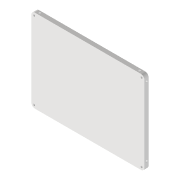
# Autodesk Inventor part: Omniscope_USBC_Illuminationunit
Saved by Autodesk Inventor 2022 (Build 260153000, 153)
## iProperties
Created: 2023-05-17
Part Number: Omniscope_USBC_Illuminationunit
Material: Generisch
Document SubType Name: Modeling
Designer: diederichbenedict
Density: 1 g/cm^3
Appearance: Vorgabe
Author: diederichbenedict
Autodesk Inventor part; units mm, degrees
ref_plane "YZ Plane" through (0, 0, 0) normal (1, 0, 0) x (0, 1, 0)
ref_plane "XZ Plane" through (0, 0, 0) normal (0, 1, 0) x (-1, 0, 0)
ref_plane "XY Plane" through (0, 0, 0) normal (0, 0, 1) x (1, 0, 0)
sketch "Skizze1" plane through (0, 0, 0) normal (0, 0, 1) x (1, 0, 0)
  line L0 (63.945, 39.8) -> (63.945, -39.8) construction
  arc A0 (63.945, 39.8) -> (60.945, 42.8) centre (60.945, 39.8) ccw construction
  line L1 (-60.945, 42.8) -> (60.945, 42.8) construction
  arc A1 (-60.945, 42.8) -> (-63.945, 39.8) centre (-60.945, 39.8) ccw construction
  line L2 (-63.945, -39.8) -> (-63.945, 39.8) construction
  arc A2 (-63.945, -39.8) -> (-60.945, -42.8) centre (-60.945, -39.8) ccw construction
  line L3 (60.945, -42.8) -> (-60.945, -42.8) construction
  arc A3 (60.945, -42.8) -> (63.945, -39.8) centre (60.945, -39.8) ccw construction
  line L4 (-63.625, -39.48) -> (-63.625, 39.48) construction
  arc A4 (-60.625, 42.48) -> (-63.625, 39.48) centre (-60.625, 39.48) ccw construction
  line L5 (-60.625, 42.48) -> (60.625, 42.48) construction
  arc A5 (63.625, 39.48) -> (60.625, 42.48) centre (60.625, 39.48) ccw construction
  line L6 (63.625, 39.48) -> (63.625, -39.48) construction
  arc A6 (60.625, -42.48) -> (63.625, -39.48) centre (60.625, -39.48) ccw construction
  line L7 (60.625, -42.48) -> (-60.625, -42.48) construction
  arc A7 (-63.625, -39.48) -> (-60.625, -42.48) centre (-60.625, -39.48) ccw construction
  line L8 (-62.625, 39.48) -> (-62.625, -39.48) construction
  arc A8 (-62.625, -39.48) -> (-60.625, -41.48) centre (-60.625, -39.48) ccw construction
  line L9 (-60.625, -41.48) -> (60.625, -41.48) construction
  arc A9 (60.625, -41.48) -> (62.625, -39.48) centre (60.625, -39.48) ccw construction
  line L10 (62.625, -39.48) -> (62.625, 39.48) construction
  arc A10 (62.625, 39.48) -> (60.625, 41.48) centre (60.625, 39.48) ccw construction
  line L11 (60.625, 41.48) -> (-60.625, 41.48) construction
  arc A11 (-60.625, 41.48) -> (-62.625, 39.48) centre (-60.625, 39.48) ccw construction
  line L12 (75.9176, 38) -> (78.9176, 41) construction
  line L13 (75.9176, 38) -> (66.9176, 38) construction
  line L14 (63.9176, 35) -> (66.9176, 38) construction
  line L15 (63.9176, 35) -> (63.9176, -34.9) construction
  line L16 (66.9176, -37.9) -> (63.9176, -34.9) construction
  line L17 (66.9176, -37.9) -> (75.9176, -37.9) construction
  line L18 (78.9176, -40.9) -> (75.9176, -37.9) construction
  line L19 (78.9176, -40.9) -> (78.9176, -45.7356) construction
  arc A12 (74.9176, -49.7356) -> (78.9176, -45.7356) centre (74.9176, -45.7356) ccw construction
  line L20 (74.9176, -49.7356) -> (-61.9244, -49.7356) construction
  arc A13 (-65.9244, -45.7356) -> (-61.9244, -49.7356) centre (-61.9244, -45.7356) ccw projected
  line L21 (-65.9244, -45.7356) -> (-65.9244, -40.9) projected
  line L22 (-62.9244, -37.9) -> (-65.9244, -40.9) projected
  line L23 (-62.9244, -37.9) -> (-58.9244, -37.9) construction
  line L24 (-55.9244, -34.9) -> (-58.9244, -37.9) construction
  line L25 (-55.9244, -34.9) -> (-55.9244, 35) construction
  line L26 (-58.9244, 38) -> (-55.9244, 35) construction
  line L27 (-58.9244, 38) -> (-62.9244, 38) construction
  line L28 (-65.9244, 41) -> (-62.9244, 38) projected
  line L29 (-65.9244, 41) -> (-65.9244, 49.0948) projected
  arc A14 (-61.9244, 53.0948) -> (-65.9244, 49.0948) centre (-61.9244, 49.0948) ccw projected
  line L30 (-61.9244, 53.0948) -> (74.9176, 53.0948) construction
  arc A15 (78.9176, 49.0948) -> (74.9176, 53.0948) centre (74.9176, 49.0948) ccw construction
  line L31 (78.9176, 49.0948) -> (78.9176, 41) construction
  circle A16 centre (-62.4244, 49.5948) radius 1.4 construction
  circle A17 centre (-62.4244, -46.2356) radius 1.4 construction
  circle A18 centre (75.4176, -46.2356) radius 1.4 construction
  circle A19 centre (75.4176, 49.5948) radius 1.5 construction
  circle A20 centre (45.2899, -42.9) radius 1.4 construction
  circle A21 centre (45.2899, 43) radius 1.4 construction
  line L32 (54.6, 38) -> (44.6, 38) construction
  line L33 (44.6, 38) -> (44.6, -37.9) construction
  line L34 (44.6, -37.9) -> (54.6, -37.9) construction
  line L35 (54.6, -37.9) -> (54.6, 38) construction
  circle A22 centre (26.5899, 43) radius 1.4 construction
  circle A23 centre (26.5899, -42.9) radius 1.4 construction
  line L36 (25.9, -37.9) -> (35.9, -37.9) construction
  line L37 (35.9, -37.9) -> (35.9, 38) construction
  line L38 (35.9, 38) -> (25.9, 38) construction
  line L39 (25.9, 38) -> (25.9, -37.9) construction
  circle A24 centre (7.8899, 43) radius 1.4 construction
  circle A25 centre (7.8899, -42.9) radius 1.4 construction
  line L40 (7.2, -37.9) -> (17.2, -37.9) construction
  line L41 (17.2, -37.9) -> (17.2, 38) construction
  line L42 (17.2, 38) -> (7.2, 38) construction
  line L43 (7.2, 38) -> (7.2, -37.9) construction
  circle A26 centre (-10.8101, 43) radius 1.4 construction
  circle A27 centre (-10.8101, -42.9) radius 1.4 construction
  line L44 (-11.5, -37.9) -> (-1.5, -37.9) construction
  line L45 (-1.5, -37.9) -> (-1.5, 38) construction
  line L46 (-1.5, 38) -> (-11.5, 38) construction
  line L47 (-11.5, 38) -> (-11.5, -37.9) construction
  circle A28 centre (-29.5101, 43) radius 1.4 construction
  circle A29 centre (-29.5101, -42.9) radius 1.4 construction
  line L48 (-30.2, -37.9) -> (-20.2, -37.9) construction
  line L49 (-20.2, -37.9) -> (-20.2, 38) construction
  line L50 (-20.2, 38) -> (-30.2, 38) construction
  line L51 (-30.2, 38) -> (-30.2, -37.9) construction
  circle A30 centre (-48.2101, 43) radius 1.4 construction
  circle A31 centre (-48.2101, -42.9) radius 1.4 construction
  line L52 (-48.9, -37.9) -> (-38.9, -37.9) construction
  line L53 (-38.9, -37.9) -> (-38.9, 38) construction
  line L54 (-38.9, 38) -> (-48.9, 38) construction
  line L55 (-48.9, 38) -> (-48.9, -37.9) construction
  line L56 (74.9176, 55.0948) -> (-61.9244, 55.0948) construction
  arc A32 (-61.9244, 55.0948) -> (-67.9244, 49.0948) centre (-61.9244, 49.0948) ccw
  line L57 (-67.9244, 49.0948) -> (-67.9244, 40.1716)
  line L58 (-67.9244, 40.1716) -> (-63.7528, 36)
  line L59 (-63.7528, 36) -> (-59.7528, 36) construction
  line L60 (-59.7528, 36) -> (-57.9244, 34.1716) construction
  line L61 (-57.9244, 34.1716) -> (-57.9244, -34.0716) construction
  line L62 (-57.9244, -34.0716) -> (-59.7528, -35.9) construction
  line L63 (-59.7528, -35.9) -> (-63.7528, -35.9) construction
  line L64 (-63.7528, -35.9) -> (-67.9244, -40.0716)
  line L65 (-67.9244, -40.0716) -> (-67.9244, -45.7356)
  arc A33 (-67.9244, -45.7356) -> (-61.9244, -51.7356) centre (-61.9244, -45.7356) ccw
  line L66 (-61.9244, -51.7356) -> (74.9176, -51.7356) construction
  arc A34 (74.9176, -51.7356) -> (80.9176, -45.7356) centre (74.9176, -45.7356) ccw construction
  line L67 (80.9176, -45.7356) -> (80.9176, -40.0716) construction
  line L68 (80.9176, -40.0716) -> (76.746, -35.9) construction
  line L69 (76.746, -35.9) -> (67.746, -35.9) construction
  line L70 (67.746, -35.9) -> (65.9176, -34.0716) construction
  line L71 (65.9176, -34.0716) -> (65.9176, 34.1716) construction
  line L72 (65.9176, 34.1716) -> (67.746, 36) construction
  line L73 (67.746, 36) -> (76.746, 36) construction
  line L74 (76.746, 36) -> (80.9176, 40.1716) construction
  line L75 (80.9176, 40.1716) -> (80.9176, 49.0948) construction
  arc A35 (80.9176, 49.0948) -> (74.9176, 55.0948) centre (74.9176, 49.0948) ccw construction
  line L76 (-61.9244, 60.0948) -> (74.9176, 60.0948) construction
  arc A36 (85.9176, 49.0948) -> (74.9176, 60.0948) centre (74.9176, 49.0948) ccw construction
  line L77 (85.9176, 49.0948) -> (85.9176, 38.1005) construction
  line L78 (85.9176, 38.1005) -> (78.8171, 31) construction
  line L79 (78.8171, 31) -> (70.9176, 31) construction
  line L80 (70.9176, 31) -> (70.9176, -30.9) construction
  line L81 (70.9176, -30.9) -> (78.8171, -30.9) construction
  line L82 (78.8171, -30.9) -> (85.9176, -38.0005) construction
  line L83 (85.9176, -38.0005) -> (85.9176, -45.7356) construction
  arc A37 (74.9176, -56.7356) -> (85.9176, -45.7356) centre (74.9176, -45.7356) ccw construction
  line L84 (74.9176, -56.7356) -> (-61.9244, -56.7356) construction
  arc A38 (-72.9244, -45.7356) -> (-61.9244, -56.7356) centre (-61.9244, -45.7356) ccw construction
  line L85 (-72.9244, -45.7356) -> (-72.9244, -38.0005) construction
  line L86 (-72.9244, -38.0005) -> (-65.8239, -30.9) construction
  line L87 (-65.8239, -30.9) -> (-62.9244, -30.9) construction
  line L88 (-62.9244, -30.9) -> (-62.9244, 31) construction
  line L89 (-62.9244, 31) -> (-65.8239, 31) construction
  line L90 (-65.8239, 31) -> (-72.9244, 38.1005) construction
  line L91 (-72.9244, 38.1005) -> (-72.9244, 49.0948) construction
  arc A39 (-61.9244, 60.0948) -> (-72.9244, 49.0948) centre (-61.9244, 49.0948) ccw construction
  line L92 (-67.9244, 60.0948) -> (80.9176, 60.0948)
  line L93 (85.9176, 55.0948) -> (85.9176, -51.7356)
  line L94 (80.9176, -56.7356) -> (-67.9244, -56.7356)
  line L95 (-72.9244, -51.7356) -> (-72.9244, 55.0948)
  arc A40 (-67.9244, 60.0948) -> (-72.9244, 55.0948) centre (-67.9244, 55.0948) ccw
  arc A41 (85.9176, 55.0948) -> (80.9176, 60.0948) centre (80.9176, 55.0948) ccw
  arc A42 (80.9176, -56.7356) -> (85.9176, -51.7356) centre (80.9176, -51.7356) ccw
  arc A43 (-72.9244, -51.7356) -> (-67.9244, -56.7356) centre (-67.9244, -51.7356) ccw
  line L96 (-60.625, -39.48) -> (60.625, -39.48)
  line L97 (60.625, -39.48) -> (60.625, 39.48)
  line L98 (60.625, 39.48) -> (-60.625, 39.48)
  line L99 (-60.625, 39.48) -> (-60.625, -39.48)
  point P0 (0, 0)
  dimension "d0" = 1
  dimension "d1" = 2
  dimension "d2" = 5
  dimension "d3" = 5
  constraints: 96 end point, 32 point on circle, 16 centre point, 8 tangent, 4 parallel, 3 equal radius, 2 horizontal, 2 perpendicular, 49 other
  measures "d0" radial gap between concentric circles of A4 A11
  measures "d1" distance between parallel lines of L30 L56
  measures "d2" distance between parallel lines of L56 L76
  measures "d3" radius of A40
extrude "Extrusion1" add sketch "Skizze1" along normal blind 1 contours L92 A41 L93 A42 L94 A43 L95 A40 | L99 L98 L97 L96
sketch "Skizze2" plane through (0, 0, 0) normal (0, 0, -1) x (-1, 0, 0)
  line L0 (67.9244, -56.7356) -> (-80.9176, -56.7356) projected
  arc A0 (67.9244, -56.7356) -> (72.9244, -51.7356) centre (67.9244, -51.7356) ccw projected
  line L1 (72.9244, 55.0948) -> (72.9244, -51.7356) projected
  arc A1 (72.9244, 55.0948) -> (67.9244, 60.0948) centre (67.9244, 55.0948) ccw projected
  line L2 (-80.9176, 60.0948) -> (67.9244, 60.0948) projected
  arc A2 (-80.9176, 60.0948) -> (-85.9176, 55.0948) centre (-80.9176, 55.0948) ccw projected
  line L3 (-85.9176, -51.7356) -> (-85.9176, 55.0948) projected
  arc A3 (-85.9176, -51.7356) -> (-80.9176, -56.7356) centre (-80.9176, -51.7356) ccw projected
  line L4 (-77.9176, 52.0948) -> (64.9244, 52.0948)
  line L5 (64.9244, 52.0948) -> (64.9244, -48.7356)
  line L6 (64.9244, -48.7356) -> (-77.9176, -48.7356)
  line L7 (-77.9176, -48.7356) -> (-77.9176, 52.0948)
  line L8 (-13.9966, 37.0948) -> (1.0034, 37.0948)
  line L9 (1.0034, 37.0948) -> (1.0034, 52.0948)
  line L10 (1.0034, 52.0948) -> (-13.9966, 52.0948)
  line L11 (-13.9966, 52.0948) -> (-13.9966, 37.0948)
  line L12 (-13.9966, 37.0948) -> (1.0034, 52.0948) construction
  line L13 (1.0034, 37.0948) -> (-13.9966, 52.0948) construction
  line L14 (-13.9966, -48.7356) -> (1.0034, -48.7356)
  line L15 (1.0034, -48.7356) -> (1.0034, 52.0948)
  line L16 (1.0034, 52.0948) -> (-13.9966, 52.0948)
  line L17 (-13.9966, 52.0948) -> (-13.9966, -48.7356)
  line L18 (-13.9966, -48.7356) -> (1.0034, 52.0948) construction
  line L19 (1.0034, -48.7356) -> (-13.9966, 52.0948) construction
  point P0 (-6.4966, 44.5948)
  point P1 (-6.4966, 1.6796)
  point P2 (1.0034, 37.0948)
  dimension "d42" = 8
  dimension "d43" = 15
  dimension "d44" = 15
  constraints: 32 end point, 4 midpoint, 4 parallel, 2 horizontal, 2 perpendicular, 1 point on line, 3 other
  measures "d42" distance between parallel lines of L3 L7
  measures "d43" distance of L10.end L9.end
  measures "d44" distance of L9.end L8.end
extrude "Extrusion2" add sketch "Skizze2" along normal blind 5 contours L0 A3 L3 A2 L2 A1 L1 A0 | L4 L9 L8 L11 | L8 L15 L6 L17
sketch "Skizze3" plane through (0, 0, -5) normal (0, 0, -1) x (-1, 0, 0)
  line L0 (67.9244, 60.0948) -> (-80.9176, 60.0948) projected
  arc A0 (-80.9176, 60.0948) -> (-85.9176, 55.0948) centre (-80.9176, 55.0948) ccw projected
  line L1 (-85.9176, 55.0948) -> (-85.9176, -51.7356) projected
  arc A1 (-85.9176, -51.7356) -> (-80.9176, -56.7356) centre (-80.9176, -51.7356) ccw projected
  line L2 (-80.9176, -56.7356) -> (67.9244, -56.7356) projected
  arc A2 (67.9244, -56.7356) -> (72.9244, -51.7356) centre (67.9244, -51.7356) ccw projected
  line L3 (72.9244, -51.7356) -> (72.9244, 55.0948) projected
  arc A3 (72.9244, 55.0948) -> (67.9244, 60.0948) centre (67.9244, 55.0948) ccw projected
  line L4 (-60.945, 43.8) -> (60.945, 43.8) projected
  arc A4 (64.945, 39.8) -> (60.945, 43.8) centre (60.945, 39.8) ccw projected
  line L5 (64.945, 39.8) -> (64.945, -39.8) projected
  arc A5 (60.945, -43.8) -> (64.945, -39.8) centre (60.945, -39.8) ccw projected
  line L6 (60.945, -43.8) -> (-60.945, -43.8) projected
  arc A6 (-64.945, -39.8) -> (-60.945, -43.8) centre (-60.945, -39.8) ccw projected
  line L7 (-64.945, -39.8) -> (-64.945, 39.8) projected
  arc A7 (-60.945, 43.8) -> (-64.945, 39.8) centre (-60.945, 39.8) ccw projected
  circle A8 centre (68.9244, -52.7356) radius 1.4
  circle A9 centre (68.9244, 56.0948) radius 1.4
  circle A10 centre (-81.9176, 56.0948) radius 1.4
  circle A11 centre (-81.9176, -52.7356) radius 1.4
  point P0 (0, 0)
  dimension "d9" = 2.8
  dimension "d10" = 2.8
  dimension "d11" = 2.8
  dimension "d12" = 2.8
  dimension "d13" = 4
  dimension "d14" = 4
  dimension "d15" = 4
  dimension "d16" = 4
  dimension "d17" = 4
  dimension "d18" = 4
  dimension "d19" = 4
  dimension "d20" = 4
  constraints: 4 centre point
  measures "d9" diameter of A8
  measures "d10" diameter of A9
  measures "d11" diameter of A10
  measures "d12" diameter of A11
  measures "d13" distance from line of A11.centre L2
  measures "d14" distance from line of L1 A11.centre
  measures "d15" horizontal distance of L1.start A10.centre
  measures "d16" distance from line of L0 A10.centre
  measures "d17" distance from line of L0 A9.centre
  measures "d18" horizontal distance of L3.end A9.centre
  measures "d19" distance from line of L2 A8.centre
  measures "d20" distance from line of L3 A8.centre
hole "Bohrung1" at (-68.9244, -52.7356, -5) at (81.9176, -52.7356, -5) at (81.9176, 56.0948, -5) at (-68.9244, 56.0948, -5) direction (0, 0, 1) diameter 2.8 end through all
sketch "Skizze4" plane through (-67.9244, 60.0948, 1) normal (0, 1, 0) x (1, 0, 0)
  circle A0 centre (143.842, -102.2347) radius 1.4 projected
  circle A1 centre (5, -102.2347) radius 1.4 projected
  line L0 (148.842, -98.2347) -> (0, -98.2347) projected
  line L1 (0, -98.2347) -> (0, -106.2347) projected
  line L2 (148.842, -106.2347) -> (0, -106.2347) projected
  line L3 (148.842, -98.2347) -> (148.842, -106.2347) projected
  circle A2 centre (3.6, 3) radius 1.4
  line L4 (0, 6) -> (148.842, 6) projected
  circle A3 centre (143.842, 3) radius 1.4
  point P0 (67.9244, 1)
  dimension "d28" = 2.8
  dimension "d29" = 3
  dimension "d30" = 2.8
  constraints: 2 centre point
  measures "d28" diameter of A2
  measures "d29" distance from line of A2.centre L4
  measures "d30" diameter of A3
extrude "Extrusion3" cut sketch "Skizze4" against normal blind 20 contours A2 | A3
sketch "Skizze5" plane through (-67.9244, -56.7356, 1) normal (0, -1, 0) x (1, 0, 0)
  circle A0 centre (143.842, -3) radius 1.4 projected
  circle A1 centre (3.6, -3) radius 1.4 projected
  point P0 (67.9244, -1)
extrude "Extrusion4" cut sketch "Skizze5" against normal blind 20
sketch "Skizze6" plane through (85.9176, -51.7356, 1) normal (1, 0, 0) x (0, 0, -1)
  circle A0 centre (-102.2347, 101.8304) radius 1.4 projected
  circle A1 centre (-102.2347, 5) radius 1.4 projected
  circle A2 centre (3, 103.2304) radius 1.4
  line L0 (6, 106.8304) -> (6, 0) projected
  circle A3 centre (3, 6.4) radius 1.4
  point P0 (1, 51.7356)
  dimension "d35" = 2.8
  dimension "d36" = 3
  dimension "d37" = 2.8
  constraints: 2 centre point
  measures "d35" diameter of A2
  measures "d36" distance from line of A2.centre L0
  measures "d37" diameter of A3
extrude "Extrusion5" cut sketch "Skizze6" against normal blind 20 contours A2 | A3
sketch "Skizze7" plane through (-72.9244, -51.7356, 1) normal (-1, 0, 0) x (0, 0, 1)
  line L0 (-4.4, -5) -> (-4.4, 3) projected
  circle A0 centre (-3, 6.4) radius 1.4 projected
  arc A1 (-1.7351, 103.8304) -> (-4.2649, 103.8304) centre (-3, 103.2304) ccw projected
  point P0 (-1, 51.7356)
extrude "Extrusion6" cut sketch "Skizze7" against normal blind 20
equation "\"d29\" = 0.5 * a3 + 0.5 * a2"
equation "\"d36\" = 0.5 * a3 + 0.5 * a2"
equation "\"a3\" = 5"
equation "\"a2\" = 1"
